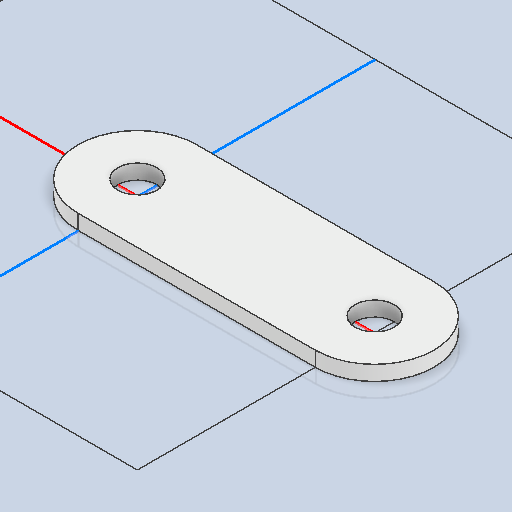
# Autodesk Inventor part: Gear Shield
Saved by Autodesk Inventor 2026 (Build 300175000, 175)
## iProperties
Created: 2025-04-12
Part Number: Gear Shield
Material: Acetal Resin, White
Document SubType Name: Modeling
Designer: avere
Density: 1.425 g/cm^3
Appearance: Smooth - White
Author: avere
Autodesk Inventor part; units mm, degrees
ref_plane "YZ Plane" through (0, 0, 0) normal (1, 0, 0) x (0, 1, 0)
ref_plane "XZ Plane" through (0, 0, 0) normal (0, 1, 0) x (-1, 0, 0)
ref_plane "XY Plane" through (0, 0, 0) normal (0, 0, 1) x (1, 0, 0)
sketch "Sketch1" plane through (0, 0, 0) normal (0, 1, 0) x (-1, 0, 0)
  circle A0 centre (0, 0) radius 2.0955
  circle A1 centre (-25.4, 0) radius 2.0955
  arc A2 (0, -6.35) -> (0, 6.35) centre (0, 0) ccw
  arc A3 (-25.4, 6.35) -> (-25.4, -6.35) centre (-25.4, 0) ccw
  line L0 (0, 6.35) -> (-25.4, 6.35)
  line L1 (-25.4, -6.35) -> (0, -6.35)
  dimension "d0" = 4.191
  dimension "d1" = 4.191
  dimension "d2" = 12.7
  dimension "d3" = 12.7
  constraints: 4 centre point, 4 end point, 4 point on circle, 3 coincident, 2 tangent
  measures "d0" diameter of A0
  measures "d1" diameter of A1
  measures "d2" diameter of A2
  measures "d3" diameter of A3
extrude "Extrusion1" add sketch "Sketch1" along normal blind 1.5875
body "Solid1"
